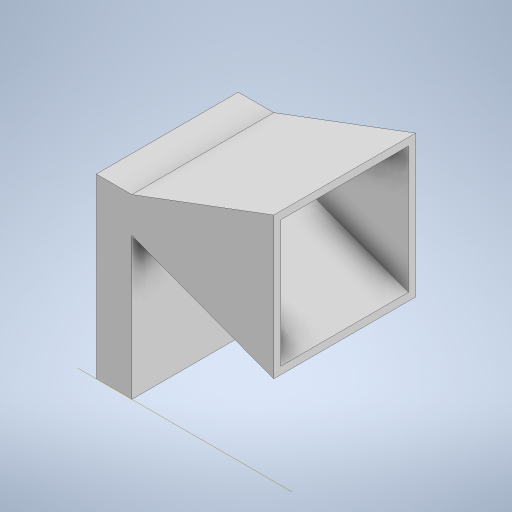
# Autodesk Inventor part: nuzzle_v1_0310
Saved by Autodesk Inventor 2023 (Build 270158000, 158)
## iProperties
Created: 2023-03-10
Part Number: nuzzle_v1_0310
Material: 一般
Document SubType Name: Modeling
Designer: USER
Density: 1 g/cm^3
Appearance: 預設
Author: USER
Autodesk Inventor part; units mm, degrees
ref_plane "YZ Plane" through (0, 0, 0) normal (1, 0, 0) x (0, 1, 0)
ref_plane "XZ Plane" through (0, 0, 0) normal (0, 1, 0) x (-1, 0, 0)
ref_plane "XY Plane" through (0, 0, 0) normal (0, 0, 1) x (1, 0, 0)
sketch "草圖1" plane through (0, 0, 0) normal (0, 1, 0) x (-1, 0, 0)
  line L0 (0, 0) -> (5, 0)
  line L1 (5, 0) -> (5, -20)
  line L2 (5, -20) -> (0, -20)
  line L3 (0, -20) -> (0, 0)
  dimension "d0" = 5
  dimension "d1" = 20
  constraints: 8 end point, 2 parallel, 1 horizontal, 1 perpendicular
  measures "d0" distance of L1.end L2.end
  measures "d1" distance of L0.end L1.end
extrude "擠出1" add sketch "草圖1" along normal blind 20
sketch "草圖3" plane through (0, 20, 0) normal (0, 1, 0) x (1, 0, 0)
  line L0 (0, 20) -> (-5, 20) projected
  line L1 (0, 0) -> (-5, 0)
  line L2 (-5, 0) -> (-5, 20)
  line L3 (-5, 20) -> (0, 20)
  line L4 (0, 20) -> (0, 0)
  constraints: 8 end point, 2 parallel, 1 horizontal, 1 perpendicular
extrude "擠出3" add sketch "草圖3" along normal blind 5
sketch "草圖4" plane through (-5, 0, 0) normal (0, 0, 1) x (1, 0, 0)
  line L0 (5, 0) -> (5, 25) projected
  line L1 (0, 25) -> (5, 25) projected
  line L2 (5, 25) -> (0, 25) projected
  line L3 (5, 25) -> (25, 32.5)
  line L4 (5, 20) -> (25, 12.5)
  line L5 (25, 12.5) -> (25, 32.5)
  line L6 (0, 0) -> (5, 0) projected
  line L7 (0, 0) -> (0, 25) projected
  line L8 (-5.1212, 0) -> (30.7273, 0) projected
  dimension "d8" = 5
  dimension "d9" = 20
  dimension "d19" = 20
  constraints: 6 end point, 1 equal length, 1 point on line, 1 vertical
  measures "d8" distance of L4.start L0.end
  measures "d9" distance of L4.end L3.end
  measures "d19" distance between parallel lines of L5 L0
extrude "擠出4" add sketch "草圖4" against normal up to surface (20 mm away) contours L0 L3 L5 L4
shell "薄殼2" thickness 1 removed faces 2 at (20, 19.1667, -6.6667) at (-1.6667, 0, -6.6667)
equation "\"d0\" = bottom_w"
equation "\"d1\" = bottom_l"
equation "\"d2\" = bottom_h"
equation "\"d6\" = nuzzle_lh"
equation "\"d8\" = nuzzle_lh"
equation "\"d9\" = 4 * nuzzle_lh"
equation "\"d15\" = nuzzle_lh"
equation "\"bottom_w\" = 5"
equation "\"bottom_l\" = 20"
equation "\"bottom_h\" = 20"
equation "\"nuzzle_lh\" = 5"
